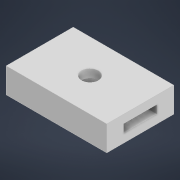
# Autodesk Inventor part: Каменъ
Saved by Autodesk Inventor 2021.2 (Build 252289000, 289)
## iProperties
Created: 2021-05-30
Part Number: Каменъ
Material: Типовые
Document SubType Name: Modeling
Designer: Admin
Density: 1 g/cm^3
Appearance: По умолчанию
Mass: 29.2854 g
Surface Area: 104.283 cm^2
Volume: 29.2854 cm^3
Author: Admin
Autodesk Inventor part; units mm, degrees
ref_plane "YZ Plane" through (0, 0, 0) normal (1, 0, 0) x (0, 1, 0)
ref_plane "XZ Plane" through (0, 0, 0) normal (0, 1, 0) x (-1, 0, 0)
ref_plane "XY Plane" through (0, 0, 0) normal (0, 0, 1) x (1, 0, 0)
sketch "Эскиз4" plane through (0, 0, 0) normal (0, 1, 0) x (-1, 0, 0)
  line L0 (30, 20) -> (-30, 20)
  line L1 (-30, 20) -> (-30, -20)
  line L2 (-30, -20) -> (30, -20)
  line L3 (30, -20) -> (30, 20)
  point P0 (0, 0)
  dimension "d16" = 40
  dimension "d17" = 20
  dimension "d18" = 60
  dimension "d19" = 30
  constraints: 8 end point, 2 parallel, 1 horizontal, 1 perpendicular
  measures "d16" distance between parallel lines of L0 L2
  measures "d17" distance from line of L0 point (0, 0)
  measures "d18" distance between parallel lines of L1 L3
  measures "d19" distance from line of L3 point (0, 0)
extrude "Выдавливание4" add sketch "Эскиз4" along normal mid plane 15
sketch "Эскиз6" plane through (30, -7.5, -20) normal (1, 0, 0) x (0, 0, -1)
  line L0 (-10, 5) -> (-30, 5)
  line L1 (-30, 5) -> (-30, 10)
  line L2 (-30, 10) -> (-10, 10)
  line L3 (-10, 10) -> (-10, 5)
  point P0 (-20, 7.5)
  dimension "d25" = 5
  dimension "d26" = 20
  dimension "d27" = 10
  dimension "d28" = 2.5
  constraints: 8 end point, 2 parallel, 1 horizontal, 1 perpendicular
  measures "d25" distance between parallel lines of L0 L2
  measures "d26" distance between parallel lines of L1 L3
  measures "d27" distance from line of point (-20, 7.5) L3
  measures "d28" distance from line of point (-20, 7.5) L0
extrude "Выдавливание5" cut sketch "Эскиз6" against normal through all
sketch "Эскиз7" plane through (0, 7.5, 0) normal (0, 1, 0) x (1, 0, 0)
  point P0 (0, 0)
  point P1 (0, 0)
  constraints: 1 coincident
hole "Отверстие2" at (0, 7.5, 0) direction (0, -1, 0) diameter 10 depth 5
equation "\"d17\" = 0.5 * d16"
equation "\"d19\" = 0.5 * d18"
equation "\"d27\" = 0.5 * d26"
equation "\"d28\" = 0.5 * d25"
